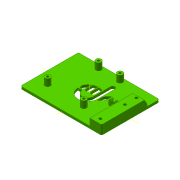
# Autodesk Inventor part: empty
Saved by Autodesk Inventor 2014 (Build 180170000, 170)
## iProperties
Created: 2015-04-13
Part Number: empty
Material: Generic
Document SubType Name: Modeling
Designer: Martin
Density: 1 g/cm^3
Appearance: Default
Author: Martin
Autodesk Inventor part; units mm, degrees
ref_plane "YZ Plane" through (0, 0, 0) normal (1, 0, 0) x (0, 1, 0)
ref_plane "XZ Plane" through (0, 0, 0) normal (0, 1, 0) x (-1, 0, 0)
ref_plane "XY Plane" through (0, 0, 0) normal (0, 0, 1) x (1, 0, 0)
sketch "sk_baseplate" plane through (0, 0, 0) normal (0, 0, 1) x (1, 0, 0)
  line L0 (0, -52.5) -> (0, 52.5) projected
  line L1 (-73.5, 0) -> (73.5, 0) projected
  line L2 (-52.5, -37.5) -> (52.5, -37.5)
  line L3 (52.5, -37.5) -> (52.5, 37.5)
  line L4 (52.5, 37.5) -> (-52.5, 37.5)
  line L5 (-52.5, 37.5) -> (-52.5, -37.5)
  line L6 (-52.5, -37.5) -> (52.5, 37.5) construction
  line L7 (52.5, -37.5) -> (-52.5, 37.5) construction
  line L8 (-12.5, 37.5) -> (-12.5, -37.5) construction
  line L9 (45, 37.5) -> (45, -37.5) construction
  line L10 (-36.6, -19.6) -> (11.6, -19.6) construction
  line L11 (11.6, -19.6) -> (11.6, 32.5) construction
  line L12 (11.6, 32.5) -> (6.5, 32.5) construction
  line L13 (6.5, 32.5) -> (-21.4, 32.5) construction
  line L14 (-21.4, 32.5) -> (-36.6, 32.5) construction
  line L15 (-36.6, 32.5) -> (-36.6, -19.6) construction
  circle A0 centre (11.6, -19.6) radius 1.5
  circle A1 centre (6.5, 32.5) radius 1.5
  circle A2 centre (-21.4, 32.5) radius 1.5
  line L16 (11.6, -18.3) -> (-36.6, -18.3) construction
  circle A3 centre (-36.6, -18.3) radius 1.5
  line L17 (37.5, -37.5) -> (52.5, -37.5)
  line L18 (52.5, -37.5) -> (52.5, 21.5)
  line L19 (52.5, 21.5) -> (37.5, 21.5)
  line L20 (37.5, 21.5) -> (37.5, -37.5)
  line L21 (37.5, -37.5) -> (52.5, 21.5) construction
  line L22 (52.5, -37.5) -> (37.5, 21.5) construction
  line L23 (27.5, -37.5) -> (27.5, 37.5) construction
  point P0 (0, 0)
  point P1 (-12.5, -19.6)
  point P2 (45, -8)
  dimension "d0" = 105
  dimension "d1" = 75
  dimension "d2" = 40
  dimension "d3" = 7.5
  dimension "d4" = 48.2
  dimension "d5" = 1.3
  dimension "d6" = 50.8
  dimension "d7" = 3
  dimension "d8" = 5
  dimension "d9" = 5.1
  dimension "d10" = 27.9
  dimension "d11" = 15
  dimension "d12" = 40
  dimension "d13" = 59
  constraints: 44 end point, 11 point on line, 8 perpendicular, 6 parallel, 5 midpoint, 4 centre point, 4 coincident, 3 equal radius, 2 collinear, 2 horizontal
  measures "d0" distance of L2.start L2.end
  measures "d1" distance of L4.end L2.start
  measures "d2" distance between parallel lines of L5 L8
  measures "d3" distance between parallel lines of L3 L9
  measures "d4" distance of L10.start L10.end
  measures "d5" distance between parallel lines of L10 L16
  measures "d6" distance between parallel lines of L14 L16
  measures "d7" diameter of A3
  measures "d8" distance between parallel lines of L4 L12
  measures "d9" distance of L11.end L12.end
  measures "d10" distance of L12.end L13.end
  measures "d11" distance of L18.end L19.end
  measures "d12" distance between parallel lines of L8 L23
  measures "d13" distance between parallel lines of L2 L19
extrude "ext_base" add sketch "sk_baseplate" along normal blind 3
extrude "ext_fingerholder" add sketch "sk_baseplate" along normal blind 12 contours L20 L1 L3 L2 | L20 L19 L3 L1
chamfer "Chamfer1" distance 6 angle 30 1 edges at (45, 21.5, 12) measured on face at (42.5, 21.5, 6)
sketch "Sketch2" plane through (0, 0, 3) normal (0, 0, 1) x (1, 0, 0)
  circle A0 centre (-36.6, -18.3) radius 1.5 projected
  circle A1 centre (-21.4, 32.5) radius 1.5 projected
  circle A2 centre (6.5, 32.5) radius 1.5 projected
  circle A3 centre (11.6, -19.6) radius 1.5 projected
  circle A4 centre (-21.4, 32.5) radius 3.5
  circle A5 centre (6.5, 32.5) radius 3.5
  circle A6 centre (11.6, -19.6) radius 3.5
  circle A7 centre (-36.6, -18.3) radius 3.5
  point P0 (0, 0)
  dimension "d21" = 2
  constraints: 4 centre point, 4 coincident, 3 equal radius
  measures "d21" radial gap between concentric circles of A1 A4
extrude "ext_pegs" add sketch "Sketch2" along normal blind 9
sketch "Sketch3" plane through (0, 0, 12) normal (0, 0, 1) x (1, 0, 0)
  line L0 (37.5, 18.0359) -> (52.5, 18.0359) projected
  line L1 (37.5, -37.5) -> (52.5, -37.5) projected
  line L2 (45, -37.5) -> (45, 18.0359) construction
  circle A0 centre (45, -31.5) radius 1.75
  circle A1 centre (45, 0.3) radius 1.75
  circle A2 centre (45, 15.3) radius 1.75
  point P0 (0, 0)
  dimension "d24" = 3.5
  dimension "d25" = 6
  dimension "d26" = 31.8
  dimension "d27" = 15
  constraints: 3 centre point, 3 point on line, 2 end point, 2 equal radius, 2 midpoint
  measures "d24" diameter of A0
  measures "d25" distance from line of L1 A0.centre
  measures "d26" distance of A1.centre A0.centre
  measures "d27" distance of A1.centre A2.centre
extrude "ext_mountholes" cut sketch "Sketch3" against normal through all
sketch "Sketch4" plane through (0, 0, 0) normal (0, 0, -1) x (-1, 0, 0)
  line L0 (0, -12.75) -> (0, 20.5)
  line L1 (-27.7979, -2.1726) -> (15.0178, -2.1726)
  circle A0 centre (0.6252, -2.1726) radius 7.1591 construction
  circle A1 centre (0.6252, -2.1726) radius 12.7273 construction
  line L2 (-12.1021, -2.1726) -> (-12.1021, 20.1001)
  line L3 (-6.5339, -2.1726) -> (-6.5339, 20.1001)
  arc A2 (-6.5339, 20.1001) -> (-12.1021, 20.1001) centre (-9.318, 20.1001) ccw
  line L4 (0.6252, -2.1726) -> (13.3524, -2.1726) construction
  arc A3 (-6.5339, -2.1726) -> (7.7842, -2.1726) centre (0.6252, -2.1726) ccw
  arc A4 (-12.1021, -2.1726) -> (13.3524, -2.1726) centre (0.6252, -2.1726) ccw
  line L5 (7.7842, -2.1726) -> (13.3524, -2.1726)
  line L6 (-4.4628, -13.8648) -> (-22.6731, -7.2369) construction
  line L7 (-13.1627, -3.7635) -> (-13.1627, 7.3728) construction
  line L8 (-13.1627, 7.3728) -> (-18.7309, 9.3995) construction
  line L9 (-18.7309, 9.3995) -> (-18.7309, -1.7369) construction
  line L10 (-18.7309, -1.7369) -> (-13.1627, -3.7635) construction
  arc A5 (-18.7309, 4.1887) -> (-13.1627, -3.7635) centre (-10.2684, 4.1887) ccw
  arc A6 (-13.1627, 1.4473) -> (-18.7309, 9.3995) centre (-21.6253, 1.4473) ccw
  line L11 (-18.7309, 4.1887) -> (-18.7309, 9.3995)
  line L12 (-13.1627, -3.7635) -> (-13.1627, 1.4473)
  line L13 (13.3524, 11.7194) -> (-6.5339, 11.7194) construction
  line L14 (-5.4733, 11.7194) -> (0.0949, 11.7194)
  line L15 (0.0949, 11.7194) -> (0.0949, -1.112)
  line L16 (0.0949, -1.112) -> (-5.4733, -1.112)
  line L17 (-5.4733, -1.112) -> (-5.4733, 11.7194)
  line L18 (1.1555, 11.7194) -> (6.7236, 11.7194)
  line L19 (6.7236, 11.7194) -> (6.7236, -1.112)
  line L20 (6.7236, -1.112) -> (1.1555, -1.112)
  line L21 (1.1555, -1.112) -> (1.1555, 11.7194)
  line L22 (13.3524, 11.7194) -> (7.7842, 11.7194)
  line L23 (7.7842, 11.7194) -> (7.7842, -1.112)
  line L24 (7.7842, -1.112) -> (13.3524, -1.112)
  line L25 (13.3524, -1.112) -> (13.3524, 11.7194)
  line L26 (7.7842, 5.3037) -> (6.7236, 5.3037) construction
  line L27 (1.1555, 5.3037) -> (0.0949, 5.3037) construction
  line L28 (-5.4733, 5.3037) -> (-6.5339, 5.3037) construction
  arc A7 (6.7236, 8.9984) -> (1.1555, 10.5436) centre (0.6252, -2.1726) ccw
  arc A8 (0.0949, 10.5436) -> (-5.4733, 8.9984) centre (0.6252, -2.1726) ccw
  line L29 (-13.1627, 7.3728) -> (-12.1021, 7.3728) construction
  line L30 (7.5616, -1.112) -> (7.5616, -2.1726) construction
  arc A9 (0.0949, 11.7093) -> (-5.4733, 10.3092) centre (0.6252, -2.1726) ccw
  arc A10 (6.7236, 10.3092) -> (1.1555, 11.7093) centre (0.6252, -2.1726) ccw
  arc A11 (13.3524, 3.3956) -> (7.7842, 9.7326) centre (0.6252, -2.1726) ccw
  arc A12 (13.3524, 3.3956) -> (-6.5339, 9.7326) centre (0.6252, -2.1726) ccw construction
  arc A13 (-5.4733, 1.6721) -> (0.0949, 1.6721) centre (-2.6892, 1.6721) ccw
  arc A14 (1.1555, 1.6721) -> (6.7236, 1.6721) centre (3.9395, 1.6721) ccw
  arc A15 (7.7842, 1.6721) -> (13.3524, 1.6721) centre (10.5683, 1.6721) ccw
  line L31 (0.6252, -14.8999) -> (13.3524, -14.8999) construction
  point P0 (0, 0)
  point P1 (13.3082, -1.112)
  point P2 (7.7842, 8.3502)
  dimension "d30" = 14.3182
  dimension "d31" = 5.5682
  dimension "d32" = 22.2727
  dimension "d33" = 0
  dimension "d34" = 5.5682
  dimension "d35" = 11.1364
  dimension "d36" = 1.5909
  dimension "d37" = 160
  dimension "d38" = 5.5682
  dimension "d39" = 1.0606
  dimension "d40" = 5.5682
  dimension "d41" = 32.0833
  dimension "d42" = 35
  constraints: 62 end point, 33 point on circle, 33 point on line, 20 tangent, 15 centre point, 11 parallel, 8 perpendicular, 6 equal length, 5 midpoint, 4 collinear, 4 concentric, 3 horizontal, 2 coincident, 2 vertical, 18 other
  measures "d30" diameter of A0
  measures "d32" distance from line of L1 A2.centre
  measures "d33" distance between parallel lines of L1 L4
  measures "d34" horizontal distance of L7.start L9.end
  measures "d35" distance of L9.end L8.end
  measures "d36" distance from line of L1 L7.start
  measures "d37" angle of L1 L6
  measures "d38" distance between parallel lines of L15 L17
  measures "d39" distance between parallel lines of L3 L17
  measures "d40" distance from line of L1 A12.start
  measures "d41" distance from line of L4.end L11
  measures "d42" distance from line of L31 A2.centre
extrude "ext_logo" cut sketch "Sketch4" against normal through all contours A3 L1 A4 | L12 A5 L1 | L1 A5 L11 A6 L12 | L1 L2 A2 L3 | A13 L17 A8 L0 | L0 A8 L15 A13 | A8 L17 A9 L0 | L0 A9 L15 A8 | A10 L19 A7 L21 | A7 L19 A14 L21 | L25 A15 L23 A11
sketch "Sketch5" plane through (0, 0, 0) normal (0, 0, -1) x (-1, 0, 0)
  circle A0 centre (-45, 0.3) radius 1.75 projected
  circle A1 centre (-45, 15.3) radius 1.75 projected
  circle A2 centre (-45, -31.5) radius 1.75 projected
  circle A3 centre (-45, 15.3) radius 3.25
  circle A4 centre (-45, 0.3) radius 3.25
  circle A5 centre (-45, -31.5) radius 3.25
  point P0 (0, 0)
  dimension "d45" = 6.5
  constraints: 3 centre point, 3 coincident, 2 equal radius
  measures "d45" diameter of A3
extrude "Extrusion6" cut sketch "Sketch5" against normal blind 4
fillet "Fillet1" radius 2 4 edges at (-52.5, -37.5, 1.5) (-52.5, 37.5, 1.5) (52.5, -37.5, 6) (52.5, 37.5, 1.5)
sketch "Sketch6" plane through (0, 0, 0) normal (0, 1, 0) x (-1, 0, 0)
  line L0 (50.5, 0) -> (-50.5, 0) projected
  line L1 (-50.5, 3) -> (-52.5, 3) projected
  line L2 (-50.5, 3) -> (50.5, 3) projected
  line L3 (52.5, 3) -> (50.5, 3) projected
  line L4 (50.5, 3) -> (52.5, 3) projected
  line L5 (50.5, 3) -> (-37.5, 3) projected
  line L6 (-37.5, 3) -> (-52.5, 3) projected
  line L7 (-18.7309, 3) -> (-13.1627, 3) projected
  line L8 (-13.1627, 3) -> (-18.7309, 3) projected
  line L9 (6.7236, 3) -> (1.1555, 3) projected
  line L10 (1.1555, 3) -> (6.7236, 3) projected
  line L11 (-5.4733, 3) -> (0.0949, 3) projected
  line L12 (0.0949, 3) -> (-5.4733, 3) projected
  line L13 (-6.5339, 3) -> (-12.1021, 3) projected
  line L14 (-12.1021, 3) -> (13.3524, 3) projected
  line L15 (13.3524, 3) -> (7.7842, 3) projected
  line L16 (7.7842, 3) -> (-6.5339, 3) projected
  line L17 (13.3524, 3) -> (7.7842, 3) projected
  line L18 (7.7842, 3) -> (13.3524, 3) projected
  line L19 (-15.1, 3) -> (-8.1, 3) projected
  line L20 (17.9, 3) -> (24.9, 3) projected
  line L21 (-10, 3) -> (-3, 3) projected
  line L22 (33.1, 3) -> (40.1, 3) projected
  line L23 (-37.5, 6) -> (-37.5, 12) projected
  line L24 (-37.5, 3) -> (-37.5, 6) projected
  line L25 (-37.5, 3) -> (-37.5, 12) projected
  line L26 (-30.5, 3) -> (-30.5, 7.8227) construction
  line L27 (-28, 3) -> (-26, 3)
  line L28 (-28, 3) -> (-26, 3)
  line L29 (-26, 3) -> (-26, 7)
  line L30 (-26, 7) -> (-28, 7)
  line L31 (-28, 7) -> (-28, 3)
  line L32 (-35, 3) -> (-33, 3)
  line L33 (-33, 3) -> (-33, 7)
  line L34 (-33, 7) -> (-35, 7)
  line L35 (-35, 7) -> (-35, 3)
  arc A0 (-28, 7) -> (-33, 7) centre (-30.5, 7) ccw construction
  arc A1 (-26, 7) -> (-35, 7) centre (-30.5, 7) ccw construction
  line L36 (-30.5, 7) -> (-33.2394, 10.5701)
  line L37 (-30.5, 7) -> (-27.7606, 10.5701)
  arc A2 (-33.2394, 10.5701) -> (-35, 7) centre (-30.5, 7) ccw
  arc A3 (-32.0219, 8.9834) -> (-33, 7) centre (-30.5, 7) ccw
  arc A4 (-28, 7) -> (-28.9781, 8.9834) centre (-30.5, 7) ccw
  arc A5 (-26, 7) -> (-27.7606, 10.5701) centre (-30.5, 7) ccw
  arc A6 (-33, 5) -> (-31, 3) centre (-31, 5) ccw
  arc A7 (-30, 3) -> (-28, 5) centre (-30, 5) ccw
  line L38 (-50.5, 3) -> (50.5, 3) projected
  point P0 (0, 0)
  dimension "d49" = 7
  dimension "d53" = 4
  dimension "d54" = 2
  dimension "d55" = 5
  dimension "d56" = 75
  dimension "d59" = 2
  constraints: 24 end point, 20 point on circle, 8 centre point, 6 tangent, 5 parallel, 4 concentric, 2 midpoint, 2 perpendicular, 2 point on line, 1 collinear, 1 horizontal, 16 other
  measures "d49" distance between parallel lines of L26 L23
  measures "d53" distance between parallel lines of L2 L30
  measures "d54" distance between parallel lines of L29 L31
  measures "d55" distance between parallel lines of L31 L33
  measures "d56" angle of L37 L36
  measures "d59" radius of A6
extrude "Extrusion7" add sketch "Sketch6" along normal mid plane 4 contours L35 L34 L33 L2 | L33 A6 L2 | A2 L36 A3 L34 | A7 L31 L2 | L31 L30 L29 L2 | A4 L37 A5 L30
ref_plane "Work Plane1" through (45, 0.3, 3.75) normal (0, 0, -1) x (-1, 0, 0)
sketch "Sketch7" plane through (0, 0, 0) normal (0, 0, -1) x (-1, 0, 0)
  circle A0 centre (-45, 0.3) radius 3.25 projected
  circle A1 centre (-45, 15.3) radius 3.25 projected
  circle A2 centre (-45, -31.5) radius 3.25 projected
  circle A3 centre (-45, 15.3) radius 2.5
  circle A4 centre (-45, 0.3) radius 2.5
  circle A5 centre (-45, -31.5) radius 2.5525
  point P0 (0, 0)
  dimension "d61" = 5
  constraints: 3 centre point, 3 coincident, 1 equal radius
  measures "d61" diameter of A3
extrude "PRINT_support" add sketch "Sketch7" against normal up to surface (3.75 mm away) contours A3 | A4 | A5
equation "\"d30\" = 0.409091 * d42"
equation "\"d31\" = d40"
equation "\"d32\" = 0.636364 * d42"
equation "\"d34\" = d40"
equation "\"d35\" = 0.318182 * d42"
equation "\"d36\" = 0.0454545 * d42"
equation "\"d38\" = d40"
body "Solid1"
